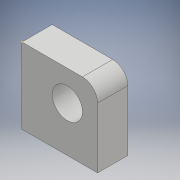
# Autodesk Inventor part: 26
Saved by Autodesk Inventor 2017 (Build 210142000, 142)
## iProperties
Part Number: 26
Material: 一般
Document SubType Name: Modeling
Designer: Brian
Density: 1 g/cm^3
Appearance: 預設
Author: Brian
Autodesk Inventor part; units mm, degrees
ref_plane "YZ Plane" through (0, 0, 0) normal (1, 0, 0) x (0, 1, 0)
ref_plane "XZ Plane" through (0, 0, 0) normal (0, 1, 0) x (-1, 0, 0)
ref_plane "XY Plane" through (0, 0, 0) normal (0, 0, 1) x (1, 0, 0)
sketch "草圖1" plane through (0, 0, 0) normal (0, 1, 0) x (-1, 0, 0)
  line L0 (0, 0) -> (-50, 0)
  line L1 (-50, 0) -> (-50, -50)
  line L2 (-50, -50) -> (0, -50)
  line L3 (0, -50) -> (0, 0)
  dimension "d0" = 50
  dimension "d1" = 50
  constraints: 8 end point, 2 parallel, 1 horizontal, 1 perpendicular
  measures "d0" distance of L2.end L0.start
  measures "d1" distance of L1.end L2.end
extrude "擠出1" add sketch "草圖1" along normal blind 20
sketch "草圖2" plane through (50, 0, -50) normal (0, 0, -1) x (-1, 0, 0)
  line L0 (50, 20) -> (0, 20) projected
  line L1 (50, 20) -> (30, 20)
  line L2 (30, 20) -> (30, 40)
  line L3 (30, 40) -> (50, 40)
  line L4 (50, 40) -> (50, 20)
  line L5 (30, 20) -> (10, 20)
  line L6 (10, 20) -> (10, 30)
  line L7 (10, 30) -> (30, 30)
  line L8 (30, 30) -> (30, 20)
  point P0 (50, 0)
  dimension "d4" = 10
  dimension "d5" = 20
  dimension "d6" = 20
  dimension "d7" = 20
  constraints: 16 end point, 4 parallel, 2 horizontal, 2 perpendicular
  measures "d4" distance of L5.end L6.end
  measures "d5" distance of L1.end L2.end
  measures "d6" distance of L2.end L3.end
  measures "d7" distance of L6.end L7.end
extrude "擠出2" add sketch "草圖2" against normal blind 10
sketch "草圖3" plane through (0, 0, -50) normal (-1, 0, 0) x (0, 0, 1)
  point P0 (50, 0)
sketch "草圖4" plane through (0, 0, -50) normal (-1, 0, 0) x (0, 0, 1)
  line L0 (50, 20) -> (0, 20) projected
  line L1 (10, 40) -> (50, 20)
  line L2 (50, 20) -> (10, 20)
  line L3 (10, 40) -> (10, 20)
  point P0 (50, 0)
  constraints: 6 end point, 1 perpendicular, 1 point on line
extrude "擠出3" add sketch "草圖4" against normal blind 10
fillet "圓角1" radius 10 1 edges at (50, 10, 0)
sketch "草圖5" plane through (0, 20, 0) normal (0, 1, 0) x (1, 0, 0)
  circle A0 centre (30, 20) radius 10
  line L0 (10, 0) -> (40, 0) projected
  line L1 (50, 10) -> (50, 50) projected
  point P0 (0, 0)
  dimension "d13" = 20
  dimension "d14" = 10
  dimension "d15" = 20
  constraints: 1 centre point
  measures "d13" diameter of A0
  measures "d14" distance edge to line of A0 L0
  measures "d15" distance from line of L1 A0.centre
extrude "擠出4" cut sketch "草圖5" against normal through all
